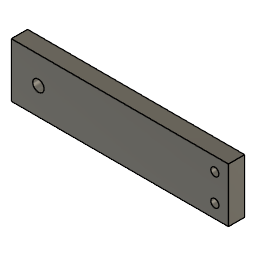
実験用台 v1 (Autodesk Fusion 360 design; units mm, degrees)
Autodesk Fusion 360 part; units mm, degrees
sketch "スケッチ1" plane through (0, 0, 0) normal (0, 0, 1) x (1, 0, 0)
  line L0 (10, -10) -> (-70, -10)
  line L1 (-70, -10) -> (-70, 0)
  line L2 (-70, 0) -> (10, 0)
  line L3 (10, 0) -> (10, -10)
  constraint horizontal L0
  constraint vertical L1
  constraint horizontal L2
  constraint vertical L3
extrude "押し出し1" add sketch "スケッチ1" along normal blind 20
sketch "スケッチ2" plane through (0, 0, 0) normal (0, 1, 0) x (-1, 0, 0)
  line L0 (-10, 0) -> (70, 0)
  line L1 (70, 0) -> (70, 20)
  line L2 (70, 20) -> (-10, 20)
  line L3 (-10, 20) -> (-10, 0)
  circle A0 centre (60, 10) radius 2.1
extrude "押し出し2" cut sketch "スケッチ2" against normal blind 10 contours A0
extrude "押し出し3" cut 1 faces at (-12.6333, -10, 10) along direction (0, 1, 0) blind 4
sketch "スケッチ3" plane through (0, 0, 0) normal (0, 1, 0) x (-1, 0, 0)
  circle A0 centre (60, 10) radius 2.1
  line L0 (-10, 0) -> (70, 0)
  line L1 (70, 0) -> (70, 20)
  line L2 (70, 20) -> (-10, 20)
  line L3 (-10, 20) -> (-10, 0)
  circle A1 centre (-5, 15) radius 1.5
  circle A2 centre (-5, 5) radius 1.5
extrude "押し出し4" cut sketch "スケッチ3" against normal blind 6 contours A1 | A2
